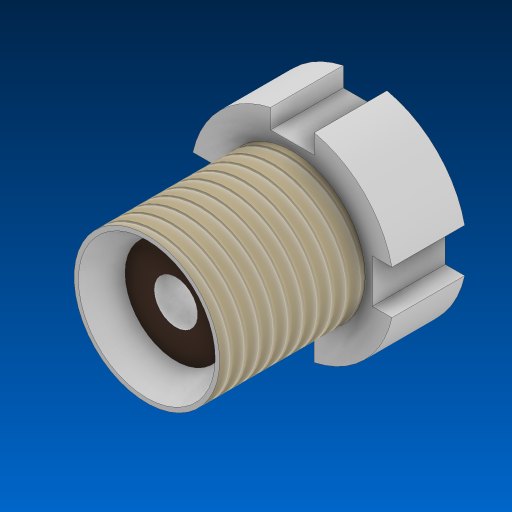
# Autodesk Inventor part: HUDSON-1-36
Saved by Autodesk Inventor 2023 (Build 270158000, 158)
## iProperties
Created: 2024-11-02
Part Number: HUDSON-1-36
Material: Generic
Document SubType Name: Modeling
Designer: CABALLERO
Density: 1 g/cm^3
Appearance: Default
Author: CABALLERO
Autodesk Inventor part; units mm, degrees
ref_plane "YZ Plane" through (0, 0, 0) normal (1, 0, 0) x (0, 1, 0)
ref_plane "XZ Plane" through (0, 0, 0) normal (0, 1, 0) x (-1, 0, 0)
ref_plane "XY Plane" through (0, 0, 0) normal (0, 0, 1) x (1, 0, 0)
sketch "Sketch1" plane through (0, 0, 0) normal (0, 0, 1) x (1, 0, 0)
  circle A0 centre (0, 0) radius 7
  dimension "d0" = 14
  constraints: 1 centre point, 1 coincident
  measures "d0" diameter of A0
extrude "Extrusion1" add sketch "Sketch1" along normal blind 5
sketch "Sketch2" plane through (0, 0, 5) normal (0, 0, 1) x (1, 0, 0)
  circle A0 centre (0, 0) radius 5
  dimension "d3" = 10
  constraints: 1 centre point, 1 coincident
  measures "d3" diameter of A0
extrude "Extrusion2" add sketch "Sketch2" along normal blind 10
thread "Thread1" size "M10x1" class "6g" standard "ANSI Metric M Profile" length 23
sketch "Sketch3" plane through (0, 0, 15) normal (0, 0, 1) x (1, 0, 0)
  point P0 (0, 0)
  point P1 (0, 0)
  constraints: 1 coincident
hole "Hole1" at (0, 0, 15) direction (0, 0, -1) diameter 7 end through all
chamfer "Chamfer1" distance 1.2 angle 60 1 edges at (0, 3.5, 15) measured on face at (4.4431, -0.5395, 15)
sketch "Sketch4" plane through (0, 0, 0) normal (0, 0, -1) x (-1, 0, 0)
  circle A0 centre (0, 0) radius 1.5
  circle A1 centre (0, 0) radius 3.5
  dimension "d18" = 3
  constraints: 2 centre point, 2 coincident
  measures "d18" diameter of A0
extrude "Extrusion3" add sketch "Sketch4" against normal blind 13
sketch "Sketch5" plane through (0, 0, 5) normal (0, 0, 1) x (1, 0, 0)
  circle A0 centre (0, 0) radius 7
  line L0 (-1.5, 8.5) -> (1.5, 8.5)
  line L1 (1.5, 8.5) -> (1.5, 5.5)
  line L2 (1.5, 5.5) -> (-1.5, 5.5)
  line L3 (-1.5, 5.5) -> (-1.5, 8.5)
  circle A1 centre (0, 0) radius 7 projected
  line L4 (-1.5, 8.5) -> (1.5, 5.5) construction
  line L5 (1.5, 8.5) -> (-1.5, 5.5) construction
  line L6 (8.5, 1.5) -> (5.5, 1.5)
  line L7 (5.5, 1.5) -> (5.5, -1.5)
  line L8 (5.5, -1.5) -> (8.5, -1.5)
  line L9 (8.5, -1.5) -> (8.5, 1.5)
  line L10 (8.5, 1.5) -> (5.5, -1.5) construction
  line L11 (5.5, 1.5) -> (8.5, -1.5) construction
  line L12 (1.5, -8.5) -> (-1.5, -8.5)
  line L13 (-1.5, -8.5) -> (-1.5, -5.5)
  line L14 (-1.5, -5.5) -> (1.5, -5.5)
  line L15 (1.5, -5.5) -> (1.5, -8.5)
  line L16 (1.5, -8.5) -> (-1.5, -5.5) construction
  line L17 (-1.5, -8.5) -> (1.5, -5.5) construction
  line L18 (-8.5, 1.5) -> (-5.5, 1.5)
  line L19 (-5.5, 1.5) -> (-5.5, -1.5)
  line L20 (-5.5, -1.5) -> (-8.5, -1.5)
  line L21 (-8.5, -1.5) -> (-8.5, 1.5)
  line L22 (-8.5, 1.5) -> (-5.5, -1.5) construction
  line L23 (-5.5, 1.5) -> (-8.5, -1.5) construction
  point P0 (0, 7)
  point P1 (7, 0)
  point P2 (0, -7)
  point P3 (-7, 0)
  dimension "d21" = 3
  dimension "d22" = 3
  dimension "d23" = 3
  dimension "d24" = 3
  dimension "d25" = 3
  dimension "d26" = 3
  dimension "d27" = 3
  dimension "d28" = 3
  constraints: 48 end point, 8 midpoint, 8 parallel, 4 horizontal, 4 perpendicular, 4 point on line, 2 point on circle, 1 centre point, 1 coincident
  measures "d21" distance of L1.end L2.end
  measures "d22" distance of L0.end L1.end
  measures "d23" distance of L8.end L7.end
  measures "d24" distance of L7.end L6.end
  measures "d25" distance of L13.end L14.end
  measures "d26" distance of L12.end L13.end
  measures "d27" distance of L19.end L20.end
  measures "d28" distance of L18.end L19.end
extrude "Extrusion4" cut sketch "Sketch5" against normal blind 13 contours A0 L8 L7 L6 | A0 L6 L9 L8 | L1 L2 L3 A0 | A0 L3 L0 L1 | L15 L12 L13 A0 | A0 L13 L14 L15 | L18 L19 L20 A0 | A0 L20 L21 L18
body "Solid1"
